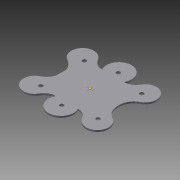
# Autodesk Inventor part: Part3
Saved by Autodesk Inventor 2015 (Build 190159000, 159)
## iProperties
Created: 2015-12-28
Part Number: Part3
Material: Generic
Document SubType Name: Modeling
Designer: Acer Aspire
Density: 1 g/cm^3
Appearance: Default
Author: Acer Aspire
Autodesk Inventor part; units mm, degrees
ref_plane "YZ Plane" through (0, 0, 0) normal (1, 0, 0) x (0, 1, 0)
ref_plane "XZ Plane" through (0, 0, 0) normal (0, 1, 0) x (-1, 0, 0)
ref_plane "XY Plane" through (0, 0, 0) normal (0, 0, 1) x (1, 0, 0)
ref_plane "Work Plane1" through (0.0967, 3, -43.9566) normal (0, 1, 0) x (1, 0, 0)
sketch "Sketch1" plane through (0.0967, 3, -43.9566) normal (0, 1, 0) x (1, 0, 0)
  line L0 (-43.4364, -51.7928) -> (-43.4364, -36.1204)
  line L1 (-43.4364, -36.1204) -> (-43.4364, -51.7928) projected
  arc A0 (-43.4364, -36.1204) -> (-54.5602, -23.1308) centre (-68.0614, -45.9505) ccw
  arc A1 (-32.3435, 0.0592) -> (-54.5602, -23.1308) centre (-47.45, -7.7054) ccw
  arc A2 (-32.3435, 0.0592) -> (-54.5602, -23.1308) centre (-47.45, -7.7054) ccw projected
  arc A3 (-32.3435, 0.0592) -> (-21.0984, -8.7493) centre (-14.9187, 10.7219) ccw
  arc A4 (-21.0984, -8.7493) -> (-16.7095, -8.8597) centre (-18.0001, 27.1171) ccw
  arc A5 (16.7095, -8.8597) -> (-16.7095, -8.8597) centre (0, 0) ccw
  arc A6 (16.7095, -8.8597) -> (21.0984, -8.7493) centre (18.0001, 27.1171) ccw
  arc A7 (21.0984, -8.7493) -> (32.3435, 0.0592) centre (14.9187, 10.7219) ccw
  arc A8 (54.5602, -23.1308) -> (32.3435, 0.0592) centre (47.45, -7.7054) ccw
  arc A9 (54.5602, -23.1308) -> (46.7947, -30.1154) centre (68.0614, -45.9505) ccw
  arc A10 (46.7947, -30.1154) -> (46.7947, -57.7978) centre (69.1023, -43.9566) ccw
  arc A11 (46.7947, -57.7978) -> (54.5602, -64.7824) centre (68.0614, -41.9626) ccw
  arc A12 (32.3435, -87.9724) -> (54.5602, -64.7824) centre (47.45, -80.2078) ccw
  arc A13 (32.3435, -87.9724) -> (21.0984, -79.1639) centre (14.9187, -98.6351) ccw
  arc A14 (21.0984, -79.1639) -> (16.7095, -79.0534) centre (18.0001, -115.0303) ccw
  arc A15 (-16.7095, -79.0534) -> (16.7095, -79.0534) centre (0, -87.9132) ccw
  arc A16 (-16.7095, -79.0534) -> (-21.0984, -79.1639) centre (-18.0001, -115.0303) ccw
  arc A17 (-21.0984, -79.1639) -> (-32.3435, -87.9724) centre (-14.9187, -98.6351) ccw
  arc A18 (-54.5602, -64.7824) -> (-32.3435, -87.9724) centre (-47.4075, -80.167) ccw
  arc A19 (-54.5602, -64.7824) -> (-43.4364, -51.7928) centre (-63.2568, -46.0771) ccw
  point P0 (-0.0967, -43.9566)
  constraints: 38 point on circle, 19 centre point, 2 end point, 1 collinear, 1 concentric, 1 tangent
extrude "Extrusion1" add sketch "Sketch1" along normal blind 2.5
sketch "Sketch2" plane through (0.0967, 5.5, -43.9566) normal (0, 1, 0) x (1, 0, 0)
  point P0 (-0.0967, -43.9566)
sketch "Sketch4" plane through (0.0967, 5.5, -43.9566) normal (0, 1, 0) x (1, 0, 0)
  point P0 (-0.0967, -43.9566)
sketch "Sketch7" plane through (0.0967, 5.5, -43.9566) normal (0, 1, 0) x (1, 0, 0)
  circle A0 centre (0.0002, -1.163) radius 3
  point P0 (-0.0967, -43.9566)
  dimension "d12" = 6
  constraints: 1 centre point
  measures "d12" diameter of A0
extrude "Extrusion5" cut sketch "Sketch7" against normal blind 3.65
sketch "Sketch8" plane through (0.0967, 5.5, -43.9566) normal (0, 1, 0) x (1, 0, 0)
  arc A0 (-16.7095, -79.0534) -> (16.7095, -79.0534) centre (0, -87.9132) ccw projected
  arc A1 (16.7095, -8.8597) -> (-16.7095, -8.8597) centre (0, 0) ccw projected
  circle A2 centre (0, -86.7513) radius 3
  point P0 (-0.0967, -43.9566)
  dimension "d15" = 87.9132
  dimension "d16" = 6
  constraints: 1 centre point
  measures "d15" distance of A0.centre A1.centre
  measures "d16" diameter of A2
extrude "Extrusion6" cut sketch "Sketch8" against normal blind 3.65
sketch "Sketch9" plane through (0.0967, 5.5, -43.9566) normal (0, 1, 0) x (1, 0, 0)
  point P0 (-0.0967, -43.9566)
sketch "Sketch21" plane through (0.0967, 5.5, -43.9566) normal (0, 1, 0) x (1, 0, 0)
  circle A0 centre (45.2429, -10.7883) radius 3
  point P0 (-0.0967, -43.9566)
  dimension "d34" = 6
  constraints: 1 centre point
  measures "d34" diameter of A0
extrude "Extrusion7" cut sketch "Sketch21" against normal blind 4.2875
sketch "Sketch22" plane through (0.0967, 5.5, -43.9566) normal (0, 1, 0) x (1, 0, 0)
  point P0 (-0.0967, -43.9566)
  point P1 (-0.0967, -43.9566)
  constraints: 1 coincident
sketch "Sketch24" plane through (0.0967, 5.5, -43.9566) normal (0, 1, 0) x (1, 0, 0)
  point P0 (-0.0967, -43.9566)
pattern_circular "Circular Pattern1" count 6 over 360 about axis through (45.3396, 5.5, -33.1683) along (0, -1, 0) of "Extrusion7"
sketch "Sketch25" plane through (0.0967, 5.5, -43.9566) normal (0, 1, 0) x (1, 0, 0)
  point P0 (-0.0967, -43.9566)
sketch "Sketch26" plane through (0.0967, 5.5, -43.9566) normal (0, 1, 0) x (1, 0, 0)
  circle A0 centre (45.18, -76.918) radius 3
  point P0 (-0.0967, -43.9566)
  dimension "d41" = 6
  constraints: 1 centre point
  measures "d41" diameter of A0
extrude "Extrusion8" cut sketch "Sketch26" against normal blind 10
sketch "Sketch27" plane through (0.0967, 3, -43.9566) normal (0, -1, 0) x (1, 0, 0)
  circle A0 centre (-41.3251, 11.0395) radius 3
  point P0 (-0.0967, 43.9566)
  dimension "d44" = 6
  constraints: 1 centre point
  measures "d44" diameter of A0
extrude "Extrusion9" cut sketch "Sketch27" against normal blind 10
sketch "Sketch28" plane through (0.0967, 3, -43.9566) normal (0, -1, 0) x (1, 0, 0)
  circle A0 centre (-41.3009, 76.9588) radius 3
  point P0 (-0.0967, 43.9566)
  dimension "d47" = 6
  constraints: 1 centre point
  measures "d47" diameter of A0
extrude "Extrusion10" cut sketch "Sketch28" against normal blind 10
body "Solid1"
